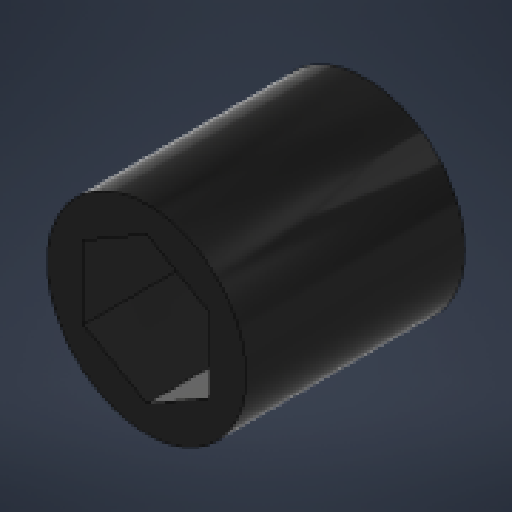
# Autodesk Inventor part: 3DPRINT,TURRET,HEX,SPACER
Saved by Autodesk Inventor 2026.1 (Build 301233020, 233B)
## iProperties
Created: 2026-02-09
Part Number: 3DPRINT,TURRET,HEX,SPACER
Material: ABS Plastic
Document SubType Name: Modeling
Designer: littl
Density: 1.06 g/cm^3
Appearance: Smooth - Black
Mass: 3.66858 g
Surface Area: 28.1201 cm^2
Volume: 3.46092 cm^3
Author: littl
Autodesk Inventor part; units mm, degrees
ref_plane "YZ Plane" through (0, 0, 0) normal (1, 0, 0) x (0, 1, 0)
ref_plane "XZ Plane" through (0, 0, 0) normal (0, 1, 0) x (-1, 0, 0)
ref_plane "XY Plane" through (0, 0, 0) normal (0, 0, 1) x (1, 0, 0)
sketch "Sketch1" plane through (0, 0, 0) normal (0, 0, 1) x (1, 0, 0)
  line L0 (-6.477, -3.7395) -> (-6.477, 3.7395)
  line L1 (-6.477, 3.7395) -> (0, 7.479)
  line L2 (0, 7.479) -> (6.477, 3.7395)
  line L3 (6.477, 3.7395) -> (6.477, -3.7395)
  line L4 (6.477, -3.7395) -> (0, -7.479)
  line L5 (0, -7.479) -> (-6.477, -3.7395)
  circle A0 centre (0, 0) radius 10.16
  dimension "d0" = 12.954
  dimension "d1" = 20.32
  constraints: 12 end point, 2 coincident, 1 centre point, 1 vertical, 13 other
  measures "d0" distance between parallel lines of L3 L0
  measures "d1" diameter of A0
extrude "Extrusion1" add sketch "Sketch1" along normal blind 22.2885
body "Solid1"
